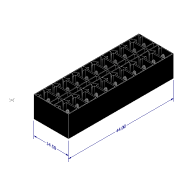
# Autodesk Inventor part: conectores
Saved by Autodesk Inventor 2022 (Build 260153000, 153)
## iProperties
Created: 2022-11-18
Part Number: conectores
Material: Generic
Document SubType Name: Modeling
Designer: ferna
Density: 1 g/cm^3
Appearance: Default
Author: ferna
Autodesk Inventor part; units mm, degrees
ref_plane "YZ Plane" through (0, 0, 0) normal (1, 0, 0) x (0, 1, 0)
ref_plane "XZ Plane" through (0, 0, 0) normal (0, 1, 0) x (-1, 0, 0)
ref_plane "XY Plane" through (0, 0, 0) normal (0, 0, 1) x (1, 0, 0)
sketch "Sketch1" plane through (0, 0, 0) normal (0, 1, 0) x (-1, 0, 0)
  line L0 (0, 0) -> (6, 0)
  line L1 (6, 0) -> (6, -3.5)
  line L2 (6, -3.5) -> (0, -3.5)
  line L3 (0, -3.5) -> (0, 0)
  line L4 (4.4594, 0) -> (4.4594, -1)
  line L5 (4.4594, -1) -> (4.6594, -1)
  line L6 (4.6594, -1) -> (4.6594, -0.7)
  line L7 (4.6594, -0.7) -> (6, 0)
  line L8 (6, -1.75) -> (5.4751, -1.75)
  line L9 (4.4594, -3.5) -> (4.4594, -2.5)
  line L10 (4.4594, -2.5) -> (4.6594, -2.5)
  line L11 (4.6594, -2.5) -> (4.6594, -2.8)
  line L12 (4.6594, -2.8) -> (6, -3.5)
  line L13 (0, 0) -> (0, 0.25)
  line L14 (0, 0.25) -> (-0.25, 0.25)
  line L15 (-0.25, 0.25) -> (6.25, 0.25)
  line L16 (6.25, 0.25) -> (6.25, -3.75)
  line L17 (6.25, -3.75) -> (-0.25, -3.75)
  line L18 (-0.25, -3.75) -> (-0.25, 0.25)
  dimension "d0" = 6
  dimension "d1" = 3.5
  dimension "d2" = 1
  dimension "d3" = 0.2
  dimension "d4" = 0.3
  dimension "d5" = 0.25
  dimension "d6" = 0.25
  dimension "d7" = 6.5
  dimension "d8" = 4
  constraints: 38 end point, 6 parallel, 5 perpendicular, 4 symmetric about line, 3 horizontal, 1 midpoint, 1 point on line
  measures "d0" distance of L1.end L2.end
  measures "d1" distance of L0.end L1.end
  measures "d2" distance of L4.start L4.end
  measures "d3" distance of L4.end L5.end
  measures "d4" distance of L5.end L6.end
  measures "d5" distance of L0.start L13.end
  measures "d6" distance of L13.end L14.end
  measures "d7" distance of L16.end L17.end
  measures "d8" distance of L15.end L16.end
extrude "Extrusion1" add sketch "Sketch1" along normal blind 8 contours L0 L7 L6 L5 L4 | L9 L10 L11 L12 L2 | L15 L16 L17 L18 L14
sketch "Sketch2" plane through (0, 0, 0) normal (0, -1, 0) x (1, 0, 0)
  line L0 (-6.25, 0.25) -> (0.25, 0.25) projected
  line L1 (0.25, 0.25) -> (0.25, -3.75) projected
  line L2 (0.25, -3.75) -> (-6.25, -3.75) projected
  line L3 (-6.25, -3.75) -> (-6.25, 0.25) projected
  point P0 (0, 0)
extrude "Extrusion2" add sketch "Sketch2" along normal blind 1
sketch "Sketch3" plane through (0, 0, 0) normal (0, 1, 0) x (1, 0, 0)
  line L0 (0, 3.5) -> (0, 0) projected
  line L1 (0, 1.75) -> (-2.2, 1.75)
  line L2 (-2.5535, 1.2613) -> (-1.8465, 1.2613)
  line L3 (-1.8465, 1.2613) -> (-1.8465, 2.2387)
  line L4 (-1.8465, 2.2387) -> (-2.5535, 2.2387)
  line L5 (-2.5535, 2.2387) -> (-2.5535, 1.2613)
  line L6 (-2.5535, 1.2613) -> (-1.8465, 2.2387) construction
  line L7 (-1.8465, 1.2613) -> (-2.5535, 2.2387) construction
  dimension "d13" = 2.2
  constraints: 14 end point, 3 midpoint, 2 horizontal, 2 parallel, 1 perpendicular
  measures "d13" distance of L1.start L1.end
extrude "Extrusion3" add sketch "Sketch3" along normal blind 7 separate body
ref_plane "Work Plane1" through (0, 7.5, 0) normal (0, 1, 0) x (1, 0, 0)
sketch "Sketch5" plane through (0, 7.5, 0) normal (0, 1, 0) x (1, 0, 0)
  line L0 (-1.8465, 1.2613) -> (-1.8465, 2.2387) projected
  line L1 (-1.8465, 1.75) -> (-2.2, 1.75)
  line L2 (-2.5535, 2.2387) -> (-2.5535, 1.2613) projected
  line L3 (-2.3447, 1.5023) -> (-2.0553, 1.5023)
  line L4 (-2.0553, 1.5023) -> (-2.0553, 1.9977)
  line L5 (-2.0553, 1.9977) -> (-2.3447, 1.9977)
  line L6 (-2.3447, 1.9977) -> (-2.3447, 1.5023)
  line L7 (-2.3447, 1.5023) -> (-2.0553, 1.9977) construction
  line L8 (-2.0553, 1.5023) -> (-2.3447, 1.9977) construction
  point P0 (0, 0)
  dimension "d17" = 0.3535
  constraints: 14 end point, 3 midpoint, 2 parallel, 2 perpendicular, 1 horizontal
  measures "d17" distance of L1.start L1.end
loft "Loft1" add profiles "Sketch5" bodies 2 section 1 edges at (-1.8465, 7, -1.75) (-2.2, 7, -2.2387) (-2.5535, 7, -1.75) (-2.2, 7, -1.2613)
sketch "Sketch6" plane through (0, -1, 0) normal (0, -1, 0) x (1, 0, 0)
  point P0 (0, 0)
  point P1 (-17.7336, -1.9744)
pattern_linear "Rectangular Pattern1" count 11 spacing 4 along (0, 0, -1) count 2 spacing 8 along (1, 0, 0) of "Extrusion1", "Extrusion2" bodies 1
pattern_linear "Rectangular Pattern2" count 11 spacing 4 along (0, 0, -1) count 2 spacing 8 along (1, 0, 0) of "Loft1", "Extrusion3" bodies 2
sketch "Sketch7" plane through (0, -1, 0) normal (0, -1, 0) x (1, 0, 0)
  line L0 (1.75, 0.25) -> (8.25, 0.25) projected
  line L1 (-6.25, -43.75) -> (0.25, -43.75) projected
  line L2 (2.6814, 0.25) -> (-0.4458, 0.25)
  line L3 (-0.4458, 0.25) -> (-0.4458, -43.75)
  line L4 (-0.4458, -43.75) -> (2.6814, -43.75)
  line L5 (2.6814, -43.75) -> (2.6814, 0.25)
  point P0 (0, 0)
  constraints: 8 end point, 2 parallel, 2 point on line, 1 horizontal, 1 perpendicular
extrude "Extrusion4" add sketch "Sketch7" against normal up to surface (1 mm away) bodies 1
sketch "Sketch8" plane through (0.25, 0, 0.25) normal (0, 1, 0) x (1, 0, 0)
  line L0 (1.5, 0) -> (8, 0)
  line L1 (0, 0) -> (0, 44)
  line L2 (1.5, 0) -> (0, 0)
  line L3 (0, 0) -> (0, 0.25)
  line L4 (0, 0.25) -> (1.5, 0.25)
  line L5 (1.5, 0.25) -> (1.5, 0)
  line L6 (-4.7094, 3.75) -> (-0.25, 3.75)
  line L7 (-0.25, 4.25) -> (-4.7094, 4.25)
  line L8 (-4.7094, 7.75) -> (-0.25, 7.75)
  line L9 (-4.7094, 11.75) -> (-0.25, 11.75)
  line L10 (-4.7094, 10.75) -> (-4.7094, 11.75)
  line L11 (-4.9094, 10.75) -> (-4.7094, 10.75)
  line L12 (-4.9094, 11.05) -> (-4.9094, 10.75)
  line L13 (-6.25, 11.75) -> (-4.9094, 11.05)
  line L14 (-6.25, 8.25) -> (-6.25, 11.75)
  line L15 (-4.9094, 8.95) -> (-6.25, 8.25)
  line L16 (-4.9094, 9.25) -> (-4.9094, 8.95)
  line L17 (-4.7094, 9.25) -> (-4.9094, 9.25)
  line L18 (-4.7094, 8.25) -> (-4.7094, 9.25)
  line L19 (-0.25, 8.25) -> (-4.7094, 8.25)
  line L20 (-0.25, 11.75) -> (-0.25, 8.25)
  line L21 (-0.25, 12.25) -> (-4.7094, 12.25)
  line L22 (-4.7094, 15.75) -> (-0.25, 15.75)
  line L23 (-0.25, 16.25) -> (-4.7094, 16.25)
  line L24 (-4.7094, 19.75) -> (-0.25, 19.75)
  line L25 (-0.25, 20.25) -> (-4.7094, 20.25)
  line L26 (-4.7094, 23.75) -> (-0.25, 23.75)
  line L27 (-4.7094, 22.75) -> (-4.7094, 23.75)
  line L28 (-4.9094, 22.75) -> (-4.7094, 22.75)
  line L29 (-4.9094, 23.05) -> (-4.9094, 22.75)
  line L30 (-6.25, 23.75) -> (-4.9094, 23.05)
  line L31 (-6.25, 20.25) -> (-6.25, 23.75)
  line L32 (-4.9094, 20.95) -> (-6.25, 20.25)
  line L33 (-4.9094, 21.25) -> (-4.9094, 20.95)
  line L34 (-4.7094, 21.25) -> (-4.9094, 21.25)
  line L35 (-4.7094, 20.25) -> (-4.7094, 21.25)
  line L36 (-0.25, 20.25) -> (-4.7094, 20.25)
  line L37 (-0.25, 23.75) -> (-0.25, 20.25)
  line L38 (-4.7094, 27.75) -> (-0.25, 27.75)
  line L39 (-4.7094, 26.75) -> (-4.7094, 27.75)
  line L40 (-4.9094, 26.75) -> (-4.7094, 26.75)
  line L41 (-4.9094, 27.05) -> (-4.9094, 26.75)
  line L42 (-6.25, 27.75) -> (-4.9094, 27.05)
  line L43 (-6.25, 24.25) -> (-6.25, 27.75)
  line L44 (-4.9094, 24.95) -> (-6.25, 24.25)
  line L45 (-4.9094, 25.25) -> (-4.9094, 24.95)
  line L46 (-4.7094, 25.25) -> (-4.9094, 25.25)
  line L47 (-4.7094, 24.25) -> (-4.7094, 25.25)
  line L48 (-0.25, 24.25) -> (-4.7094, 24.25)
  line L49 (-0.25, 27.75) -> (-0.25, 24.25)
  line L50 (-4.7094, 31.75) -> (-0.25, 31.75)
  line L51 (-4.7094, 30.75) -> (-4.7094, 31.75)
  line L52 (-4.9094, 30.75) -> (-4.7094, 30.75)
  line L53 (-4.9094, 31.05) -> (-4.9094, 30.75)
  line L54 (-6.25, 31.75) -> (-4.9094, 31.05)
  line L55 (-6.25, 28.25) -> (-6.25, 31.75)
  line L56 (-4.9094, 28.95) -> (-6.25, 28.25)
  line L57 (-4.9094, 29.25) -> (-4.9094, 28.95)
  line L58 (-4.7094, 29.25) -> (-4.9094, 29.25)
  line L59 (-4.7094, 28.25) -> (-4.7094, 29.25)
  line L60 (-0.25, 28.25) -> (-4.7094, 28.25)
  line L61 (-0.25, 31.75) -> (-0.25, 28.25)
  line L62 (-4.7094, 35.75) -> (-0.25, 35.75)
  line L63 (-4.7094, 34.75) -> (-4.7094, 35.75)
  line L64 (-4.9094, 34.75) -> (-4.7094, 34.75)
  line L65 (-4.9094, 35.05) -> (-4.9094, 34.75)
  line L66 (-6.25, 35.75) -> (-4.9094, 35.05)
  line L67 (-6.25, 32.25) -> (-6.25, 35.75)
  line L68 (-4.9094, 32.95) -> (-6.25, 32.25)
  line L69 (-4.9094, 33.25) -> (-4.9094, 32.95)
  line L70 (-4.7094, 33.25) -> (-4.9094, 33.25)
  line L71 (-4.7094, 32.25) -> (-4.7094, 33.25)
  line L72 (-0.25, 32.25) -> (-4.7094, 32.25)
  line L73 (-0.25, 35.75) -> (-0.25, 32.25)
  line L74 (-4.7094, 39.75) -> (-0.25, 39.75)
  line L75 (-4.7094, 38.75) -> (-4.7094, 39.75)
  line L76 (-4.9094, 38.75) -> (-4.7094, 38.75)
  line L77 (-4.9094, 39.05) -> (-4.9094, 38.75)
  line L78 (-6.25, 39.75) -> (-4.9094, 39.05)
  line L79 (-6.25, 36.25) -> (-6.25, 39.75)
  line L80 (-4.9094, 36.95) -> (-6.25, 36.25)
  line L81 (-4.9094, 37.25) -> (-4.9094, 36.95)
  line L82 (-4.7094, 37.25) -> (-4.9094, 37.25)
  line L83 (-4.7094, 36.25) -> (-4.7094, 37.25)
  line L84 (-0.25, 36.25) -> (-4.7094, 36.25)
  line L85 (-0.25, 39.75) -> (-0.25, 36.25)
  line L86 (-4.7094, 43.75) -> (-0.25, 43.75)
  line L87 (-4.7094, 42.75) -> (-4.7094, 43.75)
  line L88 (-4.9094, 42.75) -> (-4.7094, 42.75)
  line L89 (-4.9094, 43.05) -> (-4.9094, 42.75)
  line L90 (-6.25, 43.75) -> (-4.9094, 43.05)
  line L91 (-6.25, 40.25) -> (-6.25, 43.75)
  line L92 (-4.9094, 40.95) -> (-6.25, 40.25)
  line L93 (-4.9094, 41.25) -> (-4.9094, 40.95)
  line L94 (-4.7094, 41.25) -> (-4.9094, 41.25)
  line L95 (-4.7094, 40.25) -> (-4.7094, 41.25)
  line L96 (-0.25, 40.25) -> (-4.7094, 40.25)
  line L97 (-0.25, 43.75) -> (-0.25, 40.25)
  line L98 (1.5, 44) -> (1.5, 0)
  line L99 (1.5, 44) -> (0, 44)
  line L100 (1.5, 43.75) -> (0, 43.75)
  line L101 (0, 43.75) -> (0, 44)
  line L102 (0, 44) -> (1.5, 44)
  line L103 (1.5, 44) -> (1.5, 43.75)
  line L104 (1.5, 40.25) -> (0, 40.25)
  line L105 (0, 40.25) -> (0, 39.75)
  line L106 (0, 39.75) -> (1.5, 39.75)
  line L107 (1.5, 39.75) -> (1.5, 40.25)
  line L108 (1.5, 36.25) -> (0, 36.25)
  line L109 (0, 36.25) -> (0, 35.75)
  line L110 (0, 35.75) -> (1.5, 35.75)
  line L111 (1.5, 35.75) -> (1.5, 36.25)
  line L112 (1.5, 32.25) -> (0, 32.25)
  line L113 (0, 32.25) -> (0, 31.75)
  line L114 (0, 31.75) -> (1.5, 31.75)
  line L115 (1.5, 31.75) -> (1.5, 32.25)
  line L116 (1.5, 28.25) -> (0, 28.25)
  line L117 (0, 28.25) -> (0, 27.75)
  line L118 (0, 27.75) -> (1.5, 27.75)
  line L119 (1.5, 27.75) -> (1.5, 28.25)
  line L120 (1.5, 24.25) -> (0, 24.25)
  line L121 (0, 24.25) -> (0, 23.75)
  line L122 (0, 23.75) -> (1.5, 23.75)
  line L123 (1.5, 23.75) -> (1.5, 24.25)
  line L124 (1.5, 20.25) -> (0, 20.25)
  line L125 (0, 20.25) -> (0, 19.75)
  line L126 (0, 19.75) -> (1.5, 19.75)
  line L127 (1.5, 19.75) -> (1.5, 20.25)
  line L128 (1.5, 16.25) -> (0, 16.25)
  line L129 (0, 16.25) -> (0, 15.75)
  line L130 (0, 15.75) -> (1.5, 15.75)
  line L131 (1.5, 15.75) -> (1.5, 16.25)
  line L132 (1.5, 12.25) -> (0, 12.25)
  line L133 (0, 12.25) -> (0, 11.75)
  line L134 (0, 11.75) -> (1.5, 11.75)
  line L135 (1.5, 11.75) -> (1.5, 12.25)
  line L136 (1.5, 8.25) -> (0, 8.25)
  line L137 (0, 8.25) -> (0, 7.75)
  line L138 (0, 7.75) -> (1.5, 7.75)
  line L139 (1.5, 7.75) -> (1.5, 8.25)
  line L140 (1.5, 4.25) -> (0, 4.25)
  line L141 (0, 4.25) -> (0, 3.75)
  line L142 (0, 3.75) -> (1.5, 3.75)
  line L143 (1.5, 3.75) -> (1.5, 4.25)
  point P0 (-0.25, 0.25)
  point P1 (-2.0965, 22.4887)
  point P2 (0, 4.25)
  point P3 (0, 8.25)
  point P4 (0, 12.25)
  point P5 (0, 16.25)
  point P6 (0, 20.25)
  point P7 (0, 24.25)
  point P8 (0, 28.25)
  point P9 (0, 32.25)
  point P10 (0, 36.25)
  point P11 (0, 40.25)
  point P12 (0, 43.75)
extrude "Extrusion5" add sketch "Sketch8" along normal up to surface (8 mm away) contours L1 L4 L5 L2 | L1 L140 L98 L142 | L1 L136 L98 L138 | L1 L132 L98 L134 | L1 L128 L98 L130 | L1 L124 L98 L126 | L1 L120 L98 L122 | L1 L116 L98 L118 | L1 L112 L98 L114 | L1 L108 L98 L110 | L1 L104 L98 L106 | L1 L99 L98 L100 bodies 1
body "Solid1"
body "Solid2"
